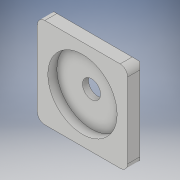
# Autodesk Inventor part: testpot
Saved by Autodesk Inventor 2017 SP1 (Build 210196100, 196)
## iProperties
Created: 2016-12-24
Part Number: testpot
Material: Generic
Document SubType Name: Modeling
Designer: wsh32
Density: 1 g/cm^3
Appearance: Default
Author: wsh32
Autodesk Inventor part; units mm, degrees
ref_plane "YZ Plane" through (0, 0, 0) normal (1, 0, 0) x (0, 1, 0)
ref_plane "XZ Plane" through (0, 0, 0) normal (0, 1, 0) x (-1, 0, 0)
ref_plane "XY Plane" through (0, 0, 0) normal (0, 0, 1) x (1, 0, 0)
sketch "Sketch1" plane through (0, 0, 0) normal (0, 0, 1) x (1, 0, 0)
  line L0 (0, 0) -> (38.1, 0)
  line L1 (38.1, 0) -> (38.1, 38.1)
  line L2 (38.1, 38.1) -> (0, 38.1)
  line L3 (0, 38.1) -> (0, 0)
  dimension "d0" = 38.1
  dimension "d1" = 38.1
  constraints: 8 end point, 2 parallel, 1 horizontal, 1 perpendicular
  measures "d0" distance of L0.start L0.end
  measures "d1" distance of L2.end L0.start
extrude "Extrusion1" add sketch "Sketch1" along normal blind 6.35
sketch "Sketch2" plane through (0, 0, 6.35) normal (0, 0, 1) x (1, 0, 0)
  line L0 (38.1, 38.1) -> (0, 38.1) construction
  line L1 (38.1, 0) -> (38.1, 38.1) construction
  line L2 (0, 38.1) -> (38.1, 0) construction
  line L3 (0, 0) -> (38.1, 38.1) construction
  point P0 (19.05, 19.05)
  constraints: 4 end point, 1 midpoint
hole "Hole1" at (19.05, 19.05, 6.35) direction (0, 0, -1) diameter 7.62 end through all counterbore diameter 29.21 counterbore depth 3.81
chamfer "Chamfer1" distance 1.27 angle 45 4 edges at (38.1, 19.05, 0) (19.05, 38.1, 0) (0, 19.05, 0) (19.05, 0, 0)
fillet "Fillet1" radius 3.175 4 edges at (38.1, 38.1, 3.81) (0, 38.1, 3.81) (38.1, 0, 3.81) (0, 0, 3.81)
body "Solid1"
